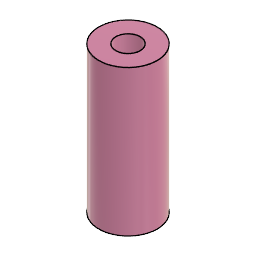
Mitoot 2804 Encoder Mount v14 (encoder magnet pin) (Autodesk Fusion 360 design; units mm, degrees)
Autodesk Fusion 360 part; units mm, degrees
sketch "Sketch1" plane through (0, 0, 0) normal (0, 0, 1) x (1, 0, 0)
  line L0 (6.75, -6.75) -> (-6.75, -6.75) construction
  line L1 (-6.75, -6.75) -> (-6.75, 6.75) construction
  line L2 (-6.75, 6.75) -> (6.75, 6.75) construction
  line L3 (6.75, 6.75) -> (6.75, -6.75) construction
  line L4 (6.75, -6.75) -> (-6.75, 6.75) construction
  line L5 (-6.75, -6.75) -> (6.75, 6.75) construction
  line L6 (8.5, -8.5) -> (-8.5, -8.5) construction
  line L7 (-8.5, -8.5) -> (-8.5, 8.5) construction
  line L8 (-8.5, 8.5) -> (8.5, 8.5) construction
  line L9 (8.5, 8.5) -> (8.5, -8.5) construction
  line L10 (8.5, -8.5) -> (-8.5, 8.5) construction
  line L11 (-8.5, -8.5) -> (8.5, 8.5) construction
  line L12 (-11.5, 11.5) -> (11.5, 11.5)
  line L13 (11.5, 11.5) -> (11.5, -11.5)
  line L14 (11.5, -11.5) -> (-11.5, -11.5)
  line L15 (-11.5, -11.5) -> (-11.5, 11.5)
  line L16 (-6.5, 6.5) -> (6.5, 6.5)
  line L17 (6.5, 6.5) -> (6.5, -6.5)
  line L18 (6.5, -6.5) -> (-6.5, -6.5)
  line L19 (-6.5, -6.5) -> (-6.5, 6.5)
  line L20 (-6.5, 6.5) -> (6.5, -6.5) construction
  line L21 (6.5, 6.5) -> (-6.5, -6.5) construction
  line L22 (0, 0) -> (11.5, 0)
  line L23 (0, 0) -> (0, -11.5)
  dimension "d1" = 13.5
  dimension "d2" = 17
  dimension "d3" = -3
  dimension "d20" = 13
  constraint horizontal L0
  constraint perpendicular L0 L1
  constraint parallel L0 L2
  constraint parallel L1 L3
  constraint coincident L4 L22.start
  constraint coincident L5 L22.start
  constraint coincident L22.start L23.start
  constraint equal L2 L3
  constraint horizontal L6
  constraint perpendicular L6 L7
  constraint parallel L6 L8
  constraint parallel L7 L9
  constraint coincident L10 L22.start
  constraint coincident L11 L22.start
  constraint equal L8 L9
  constraint horizontal L16
  constraint perpendicular L16 L17
  constraint parallel L16 L18
  constraint parallel L17 L19
  constraint coincident L20 L22.start
  constraint coincident L21 L22.start
  constraint equal L17 L18
  constraint midpoint L13 L22.end
  constraint midpoint L14 L23.end
  measures "d1" distance of L0.end L1.end
  measures "d2" distance of L6.end L7.end
  measures "d20" distance of L17.end L18.end
extrude "Extrude1" add sketch "Sketch1" along normal blind 3 contours L13 L14 L17 L18 L22 L23 | L17 L18 L22 L23 makes body 1
hole "Hole1" at (6.75, -6.75, 0) direction (0, 0, 1) diameter 2.15 end through all bodies 1
extrude "Extrude2" add sketch "Sketch1" against normal blind 3 separate body contours L13 L14 L17 L18 L22 L23 | L17 L18 L22 L23 makes body 2
hole "Hole2" at (8.5, -8.5, 0) direction (0, 0, -1) diameter 2.65 end through all bodies 2
extrude "Extrude3" add sketch "Sketch1" along normal mid plane 0.8 separate body contours L13 L14 L17 L18 L22 L23 | L17 L18 L22 L23 makes body 3
extrude "Extrude7" cut sketch "Sketch1" along normal through all and the other way through all contours L16 L17 L18 L19 L22 L23 | L17 L18 L22 L23 bodies 3
fillet "Fillet2" radius 1 1 edges at (6.5, -6.5, 0) on bodies 3
extrude "Extrude4" add sketch "Sketch1" along normal up to surface (3 mm away) and the other way up to surface (3 mm away) separate body contours L13 L14 L17 L18 L22 L23 | L17 L18 L22 L23 makes body 4
combine "Combine1" operation cut target body 4 tool bodies 1 2 makes body 5 at (6.8036, -5.6763, 1)
combine "Combine2" operation add target body 3 tool bodies 4 5
fillet "Fillet3" radius 1 2 edges at (7.2647, -8.0209, -3) (7.7523, -6.3613, 3) on bodies 3
fillet "Fillet4" radius 3 1 edges at (11.5, -11.5, 0) on bodies 3
mirror "Mirror1" about plane through (6.5, 0, 0) normal (0, 1, 0) of bodies 3 3 merged
mirror "Mirror2" about plane through (0, 6.5, 0) normal (-1, 0, 0) of bodies 3 3 merged
split "Split1" by plane through (0, 0, 0) normal (0, 0, 1) bodies 3 makes body 6 at (-1.992, 10.1653, 0.4)
sketch "Sketch2" plane through (0, 0, 0) normal (0, 0, 1) x (1, 0, 0)
  circle A0 centre (0, 0) radius 2.4
  circle A1 centre (0, 0) radius 2.1
  dimension "d39" = 4.8
  dimension "d40" = 4.2
  constraint coincident A0.centre A1.centre
  measures "d39" diameter of A0
  measures "d40" diameter of A1
extrude "Extrude8" add sketch "Sketch2" along normal blind 12 separate body contours A0 | A1 makes body 7
extrude "Extrude9" cut sketch "Sketch2" along normal blind 2 contours A1 bodies 7
hole "Hole3" at (0, 0, 2) direction (0, 0, 1) diameter 2 end through all bodies 7
hidden bodies 3 6
